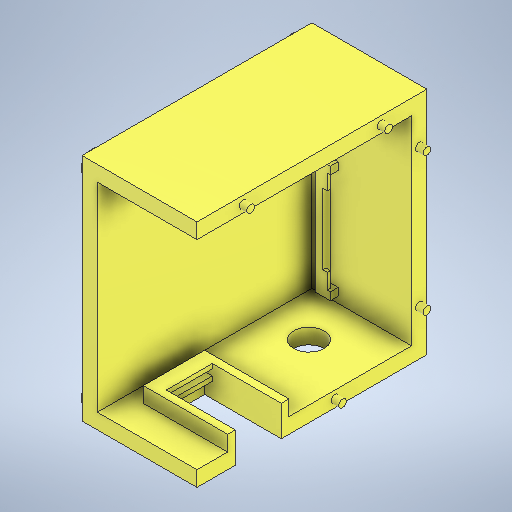
# Autodesk Inventor part: vraagblok
Saved by Autodesk Inventor 2025 (Build 290162000, 162)
## iProperties
Created: 2024-05-27
Part Number: vraagblok
Material: Generic
Document SubType Name: Modeling
Designer: wardv
Density: 1 g/cm^3
Appearance: Default
Author: wardv
Autodesk Inventor part; units mm, degrees
ref_plane "YZ Plane" through (0, 0, 0) normal (1, 0, 0) x (0, 1, 0)
ref_plane "XZ Plane" through (0, 0, 0) normal (0, 1, 0) x (-1, 0, 0)
ref_plane "XY Plane" through (0, 0, 0) normal (0, 0, 1) x (1, 0, 0)
sketch "Sketch1" plane through (0, 0, 0) normal (0, 0, 1) x (1, 0, 0)
  line L0 (0, 0) -> (75, 0)
  line L1 (75, 0) -> (75, 150)
  line L2 (75, 150) -> (0, 150)
  line L3 (0, 150) -> (0, 0)
  dimension "d0" = 75
  dimension "d1" = 150
  constraints: 8 end point, 2 parallel, 1 horizontal, 1 perpendicular
  measures "d0" distance of L2.end L1.end
  measures "d1" distance of L0.end L1.end
extrude "Extrusion1" add sketch "Sketch1" along normal blind 10
sketch "Sketch2" plane through (0, 0, 10) normal (0, 0, 1) x (1, 0, 0)
  line L0 (17, 90) -> (17, 14)
  line L1 (17, 14) -> (27, 14)
  line L2 (27, 14) -> (27, 19)
  line L3 (27, 19) -> (22, 19)
  line L4 (22, 19) -> (22, 85)
  line L5 (22, 85) -> (27, 85)
  line L6 (27, 85) -> (27, 90)
  line L7 (27, 90) -> (17, 90)
  line L8 (75, 0) -> (75, 150) projected
  line L9 (75, 150) -> (0, 150) projected
  point P0 (0, 0)
  dimension "d4" = 76
  dimension "d5" = 10
  dimension "d6" = 5
  dimension "d7" = 66
  dimension "d8" = 53
  dimension "d9" = 5
  dimension "d10" = 60
  constraints: 16 end point, 6 perpendicular, 2 point on line, 1 vertical
  measures "d4" distance of L0.start L0.end
  measures "d5" distance of L0.end L1.end
  measures "d6" distance of L1.end L2.end
  measures "d7" distance of L3.end L4.end
  measures "d8" distance between parallel lines of L8 L4
  measures "d9" distance between parallel lines of L4 L0
  measures "d10" distance between parallel lines of L9 L7
extrude "Extrusion2" add sketch "Sketch2" along normal blind 5
sketch "Sketch3" plane through (22, 19, 10) normal (1, 0, 0) x (0, 0, -1)
  line L0 (-5, 0) -> (-5, 66) projected
  line L1 (-5, 66) -> (-3, 66)
  line L2 (-3, 66) -> (-3, 56)
  line L3 (-3, 56) -> (-5, 56)
  line L4 (-5, 56) -> (-5, 66)
  line L5 (-5, 0) -> (-3, 0)
  line L6 (-3, 0) -> (-3, 10)
  line L7 (-3, 10) -> (-5, 10)
  line L8 (-5, 10) -> (-5, 0)
  point P0 (10, -19)
  point P1 (-5, 10)
  point P2 (-5, 56)
  dimension "d13" = 2
  dimension "d14" = 10
  dimension "d15" = 10
  dimension "d73" = 2
  constraints: 16 end point, 4 parallel, 2 horizontal, 2 perpendicular
  measures "d13" distance of L2.end L3.end
  measures "d14" distance of L1.end L2.end
  measures "d15" distance of L5.end L6.end
  measures "d73" distance of L6.end L7.end
extrude "Extrusion3" add sketch "Sketch3" along normal blind 3
sketch "Sketch4" plane through (0, 0, 10) normal (0, 0, 1) x (1, 0, 0)
  line L0 (75, 0) -> (75, 150) projected
  line L1 (75, 140) -> (10, 140)
  line L2 (10, 140) -> (10, 10)
  line L3 (10, 10) -> (75, 10)
  line L4 (75, 150) -> (0, 150) projected
  line L5 (0, 150) -> (0, 0) projected
  line L6 (0, 0) -> (75, 0) projected
  dimension "d18" = 10
  dimension "d19" = 10
  dimension "d20" = 10
  constraints: 6 end point, 2 perpendicular, 2 point on line, 1 horizontal
  measures "d18" distance between parallel lines of L4 L1
  measures "d19" distance between parallel lines of L5 L2
  measures "d20" distance between parallel lines of L6 L3
extrude "Extrusion4" add sketch "Sketch4" along normal blind 140 contours L6 L5 L4 L0 L1 L2 L3
sketch "Sketch5" plane through (0, 0, 0) normal (-1, 0, 0) x (0, 0, 1)
  line L0 (90.0447, 124.5126) -> (90.0447, 94.5126)
  line L1 (90.0447, 94.5126) -> (109.0447, 94.5126)
  line L2 (109.0447, 94.5126) -> (109.0447, 64.5126)
  line L3 (109.0447, 64.5126) -> (90.0447, 64.5126)
  line L4 (90.0447, 64.5126) -> (90.0447, 77.5126)
  line L5 (90.0447, 77.5126) -> (76.4377, 86.2941)
  line L6 (76.4377, 86.2941) -> (46.4377, 86.2941)
  line L7 (46.4377, 86.2941) -> (46.4377, 56.2941)
  line L8 (46.4377, 56.2941) -> (65.4377, 56.2941)
  line L9 (65.4377, 56.2941) -> (65.4377, 37.2941)
  line L10 (65.4377, 37.2941) -> (77.4951, 29.5126)
  line L11 (77.4951, 29.5126) -> (118.4951, 29.5126)
  line L12 (118.4951, 29.5126) -> (135, 48.5)
  line L13 (135, 48.5) -> (135, 111.5)
  line L14 (135, 111.5) -> (120.0447, 124.5)
  line L15 (120.0447, 124.5) -> (90.0447, 124.5126)
  line L16 (0, 0) -> (150, 0) projected
  line L17 (150, 150) -> (150, 0) projected
  line L18 (36.4377, 86) -> (17.4377, 86)
  line L19 (17.4377, 86) -> (17.4377, 56)
  line L20 (17.4377, 56) -> (36.4377, 56)
  line L21 (36.4377, 56) -> (36.4377, 86)
  line L22 (10, 140) -> (150, 140) projected
  circle A0 centre (140, 140) radius 7.5
  line L23 (10, 10) -> (150, 10) projected
  circle A1 centre (140, 10) radius 7.5
  circle A2 centre (10, 140) radius 7.5
  line L24 (10, 10) -> (10, 140) projected
  circle A3 centre (10, 10) radius 7.5
  point P0 (99.5447, 64.5126)
  point P1 (135, 80)
  point P2 (26.9377, 56)
  dimension "d43" = 30
  dimension "d44" = 19
  dimension "d45" = 30
  dimension "d46" = 13
  dimension "d47" = 30
  dimension "d48" = 30
  dimension "d49" = 19
  dimension "d50" = 19
  dimension "d51" = 41
  dimension "d52" = 63
  dimension "d53" = 13
  dimension "d56" = 35
  dimension "d57" = 95
  dimension "d58" = 30
  dimension "d59" = 80
  dimension "d60" = 25.9553
  dimension "d61" = 15
  dimension "d62" = 19
  dimension "d63" = 10
  dimension "d67" = 15
  dimension "d68" = 15
  dimension "d69" = 15
  dimension "d70" = 15
  dimension "d71" = 10
  dimension "d72" = 10
  dimension "d112" = 56
  dimension "d113" = 30
  constraints: 40 end point, 8 perpendicular, 6 parallel, 5 point on line, 4 centre point, 3 midpoint, 2 coincident, 1 horizontal, 1 vertical
  measures "d43" distance of L0.start L0.end
  measures "d44" distance of L0.end L1.end
  measures "d45" distance of L1.end L2.end
  measures "d46" distance of L3.end L4.end
  measures "d47" distance of L5.end L6.end
  measures "d48" distance of L6.end L7.end
  measures "d49" distance of L7.end L8.end
  measures "d50" distance of L8.end L9.end
  measures "d51" distance of L10.end L11.end
  measures "d52" distance of L12.end L13.end
  measures "d53" vertical distance of L13.end L14.end
  measures "d56" distance from line of point (99.545, 64.513) L11
  measures "d57" distance of L11.end L14.end
  measures "d58" distance of L14.end L0.start
  measures "d59" distance from line of L16 point (135, 80)
  measures "d60" distance between parallel lines of L2 L13
  measures "d61" distance between parallel lines of L17 L13
  measures "d62" distance of L20.end L19.end
  measures "d63" distance between parallel lines of L21 L7
  measures "d67" diameter of A0
  measures "d68" diameter of A1
  measures "d69" diameter of A2
  measures "d70" diameter of A3
  measures "d71" distance of L23.end A1.centre
  measures "d72" distance from line of L17 A0.centre
  measures "d112" distance from line of L16 point (26.938, 56)
  measures "d113" distance of L18.end L19.end
extrude "Extrusion5" add sketch "Sketch5" along normal blind 3 contours L15 L14 L13 L12 L11 L10 L9 L8 L7 L6 L5 L4 L3 L2 L1 L0 | A0 L22 | L22 A0 | A1 L23 | L23 A1 | A2 L24 L22 | L22 L24 A2 | A3 L24 L23 | L23 L24 A3 | L21 L20 L19 L18
sketch "Sketch8" plane through (10, 10, 10) normal (0, 1, 0) x (1, 0, 0)
  line L0 (65, 0) -> (65, -140) projected
  line L1 (65, -115) -> (15, -115)
  line L2 (15, -115) -> (15, -85)
  line L3 (15, -85) -> (65, -85)
  line L4 (65, -115) -> (65, -120)
  line L5 (65, -120) -> (10, -120)
  line L6 (10, -120) -> (10, -80)
  line L7 (10, -80) -> (65, -80)
  line L8 (-10, -140) -> (65, -140) projected
  point P0 (-10, 10)
  dimension "d74" = 30
  dimension "d75" = 50
  dimension "d76" = 5
  dimension "d77" = 55
  dimension "d78" = 40
  dimension "d111" = 20
  constraints: 14 end point, 5 perpendicular, 4 point on line, 1 horizontal
  measures "d74" distance of L1.end L2.end
  measures "d75" distance of L1.start L1.end
  measures "d76" distance of L1.start L4.end
  measures "d77" distance of L4.end L5.end
  measures "d78" distance of L5.end L6.end
  measures "d111" distance between parallel lines of L8 L5
extrude "Extrusion6" add sketch "Sketch8" along normal blind 10 contours L0 L3 L2 L1 L5 L6 L7
sketch "Sketch10" plane through (25, 10, 125) normal (0, 1, 0) x (1, 0, 0)
  line L0 (50, 30) -> (50, 0) projected
  line L1 (0, 30) -> (50, 30) projected
  line L2 (50, 0) -> (0, 0)
  line L3 (0, 0) -> (0, 30)
  line L4 (0, 30) -> (50, 30)
  line L5 (50, 30) -> (50, 0)
  point P0 (-25, 125)
  constraints: 8 end point, 2 parallel, 1 horizontal, 1 perpendicular
extrude "Extrusion7" cut sketch "Sketch10" against normal blind 10
sketch "Sketch11" plane through (25, 0, 95) normal (1, 0, 0) x (0, 0, -1)
  line L0 (85, 10) -> (-55, 10) projected
  line L1 (-29.957, 10) -> (0.043, 10)
  line L2 (0.043, 10) -> (0.043, 13)
  line L3 (0.043, 13) -> (-29.957, 13)
  line L4 (-29.957, 13) -> (-29.957, 10)
  line L5 (-30, 20) -> (0, 20) projected
  line L6 (-30, 20) -> (0, 20)
  line L7 (0, 20) -> (0, 17)
  line L8 (0, 17) -> (-30, 17)
  line L9 (-30, 17) -> (-30, 20)
  point P0 (95, 0)
  dimension "d83" = 30
  dimension "d84" = 30
  dimension "d85" = 3
  dimension "d86" = 3
  constraints: 16 end point, 4 parallel, 2 horizontal, 2 perpendicular, 1 point on line
  measures "d83" distance of L3.end L2.end
  measures "d84" distance of L7.end L8.end
  measures "d85" distance between parallel lines of L0 L3
  measures "d86" distance between parallel lines of L5 L8
extrude "Extrusion8" add sketch "Sketch11" along normal blind 5
sketch "Sketch12" plane through (75, 0, 0) normal (1, 0, 0) x (0, 0, -1)
  circle A0 centre (-5, 30) radius 2.5
  circle A1 centre (-5, 120) radius 2.5
  circle A2 centre (-120, 145) radius 2.5
  circle A3 centre (-30, 145) radius 2.5
  circle A4 centre (-60, 5) radius 2.5
  line L0 (-150, 140) -> (-150, 150) projected
  line L1 (0, 150) -> (-150, 150) projected
  line L2 (0, 0) -> (0, 150) projected
  line L3 (0, 0) -> (-95, 0) projected
  line L4 (-10, 10) -> (-90, 10) projected
  point P0 (-150, 145)
  dimension "d89" = 5
  dimension "d90" = 5
  dimension "d91" = 5
  dimension "d92" = 5
  dimension "d93" = 5
  dimension "d94" = 30
  dimension "d95" = 5
  dimension "d96" = 30
  dimension "d97" = 5
  dimension "d98" = 5
  dimension "d99" = 30
  dimension "d100" = 30
  dimension "d101" = 5
  dimension "d102" = 5
  dimension "d103" = 60
  constraints: 5 centre point, 1 midpoint
  measures "d89" diameter of A0
  measures "d90" diameter of A1
  measures "d91" diameter of A2
  measures "d92" diameter of A3
  measures "d93" diameter of A4
  measures "d94" distance of point (-150, 145) A2.centre
  measures "d95" distance from line of L1 A2.centre
  measures "d96" distance from line of L2 A3.centre
  measures "d97" distance from line of L1 A3.centre
  measures "d98" distance from line of L2 A1.centre
  measures "d99" distance from line of L1 A1.centre
  measures "d100" distance from line of L3 A0.centre
  measures "d101" distance from line of L2 A0.centre
  measures "d102" distance from line of L4 A4.centre
  measures "d103" distance from line of L2 A4.centre
sketch "Sketch13" plane through (0, 0, 0) normal (0, -1, 0) x (1, 0, 0)
  circle A0 centre (38, 40) radius 10
  line L0 (75, 0) -> (75, 95) projected
  line L1 (0, 0) -> (75, 0) projected
  point P0 (37.5, 0)
  dimension "d106" = 20
  dimension "d107" = 37
  dimension "d108" = 40
  constraints: 1 centre point, 1 midpoint
  measures "d106" diameter of A0
  measures "d107" distance from line of L0 A0.centre
  measures "d108" vertical distance of point (37.5, 0) A0.centre
extrude "Extrusion9" add sketch "Sketch12" along normal blind 5
extrude "Extrusion10" cut sketch "Sketch13" against normal blind 10
body "Solid1"
